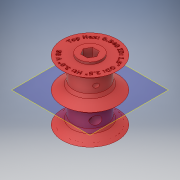
# Autodesk Inventor part: spoolV08
Saved by Autodesk Inventor 2019.4 (Build 234330000, 330)
## iProperties
Created: 2019-02-25
Part Number: spoolV08
Material: PC/ABS Plastic
Document SubType Name: Modeling
Designer: steele
Density: 0.357273 g/cm^3
Appearance: Smooth - Red
holeForString: 0.200 in
stringDiameter: 0.120 in
clearanceForString: 0.080 in
clearanceForHexShaft: 0.040 in
spoolInteriorDiameter: 1.500 in
spoolInteriroRadius: 0.750 in
spoolExteriorDiameter: 2.500 in
spoolExteriorRadius: 1.250 in
hexHoleChamfer: 0.063 in
stringHoleCenterFromHexShaft: 0.370 in
textCircleDiameter: 1.875 in
textHeight: 0.180 in
textDepth: 0.050 in
Author: steele
Autodesk Inventor part; units mm, degrees
(part 1 of 2)
ref_plane "XZ Plane" through (0, 0, 0) normal (0, 1, 0) x (-1, 0, 0)
sketch "Sketch15" plane through (0, 0, 0) normal (0, 0, 1) x (1, 0, 0)
  line L0 (31.75, 0) -> (31.75, 69.85) construction
  line L1 (12.065, 0) -> (31.75, 0)
  line L2 (13.335, 69.85) -> (31.75, 69.85)
  line L3 (19.05, 0) -> (19.05, 69.85) construction
  line L4 (0, 69.85) -> (0, 0)
  line L5 (19.05, 17.4625) -> (31.75, 17.4625) construction
  line L6 (31.75, 0) -> (19.05, 7.3323)
  line L7 (31.75, 34.925) -> (19.05, 27.5927)
  line L8 (19.05, 27.5927) -> (31.75, 27.5927) construction
  line L9 (19.05, 27.5927) -> (19.05, 7.3323)
  line L10 (31.75, 34.925) -> (19.05, 42.2573)
  line L11 (19.05, 42.2573) -> (19.05, 62.5177)
  line L12 (19.05, 62.5177) -> (31.75, 69.85)
  line L13 (31.75, 34.925) -> (19.05, 34.925) construction
  line L14 (19.05, 62.5177) -> (31.75, 62.5177) construction
  line L15 (0, 69.85) -> (0, 72.39)
  line L16 (0, 72.39) -> (13.335, 72.39)
  line L17 (13.335, 72.39) -> (13.335, 69.85)
  line L18 (0, 0) -> (0, -2.54)
  line L19 (0, -2.54) -> (12.065, -2.54)
  line L20 (12.065, -2.54) -> (12.065, 0)
  dimension "d85" = 31.75
  dimension "d86" = 69.85
  dimension "d87" = 19.05
  dimension "d88" = 31.75
  dimension "d89" = 34.925
  dimension "centerLineForSpool" = 17.4625
  dimension "d93" = 30
  dimension "d94" = 30
  dimension "d95" = 30
  dimension "d96" = 30
  dimension "d149" = 2.54
  dimension "d150" = 13.335
  dimension "d151" = 2.54
  dimension "d152" = 12.065
  constraints: 42 end point, 10 point on line, 5 perpendicular, 3 horizontal, 3 vertical, 2 midpoint, 1 collinear, 1 parallel
  measures "d85" distance from line of L4.end L0
  measures "d86" distance of L0.start L0.end
  measures "d87" distance from line of L3 L4.end
  measures "d88" distance of L4.start L0.end
  measures "d89" distance from line of L7.start L1
  measures "centerLineForSpool" distance from line of L5.start L1
  measures "d93" angle of L6 L1
  measures "d94" angle of L7 L8
  measures "d95" angle of L10 L13
  measures "d96" angle of L12 L14
  measures "d149" distance between parallel lines of L16 L2
  measures "d150" distance between parallel lines of L17 L15
  measures "d151" distance from line of L4.end L19
  measures "d152" distance between parallel lines of L20 L18
revolve "Revolution2" add sketch "Sketch15" angle 360 about axis through (0, 69.85, 0) along (0, -1, 0)
sketch "Sketch16" plane through (0, 0, 0) normal (0, -1, 0) x (1, 0, 0)
  line L0 (-7.9189, 0) -> (-3.9595, 6.858)
  line L1 (-3.9595, 6.858) -> (3.9595, 6.858)
  line L2 (3.9595, 6.858) -> (7.9189, 0)
  line L3 (7.9189, 0) -> (3.9595, -6.858)
  line L4 (3.9595, -6.858) -> (-3.9595, -6.858)
  line L5 (-3.9595, -6.858) -> (-7.9189, 0)
  point P0 (0, 0)
  point P1 (0, 0)
  dimension "d103" = 13.716
  constraints: 12 end point, 1 coincident, 1 horizontal, 13 other
  measures "d103" distance between parallel lines of L1 L4
extrude "Extrusion11" cut sketch "Sketch16" against normal through all
sketch "Sketch17" plane through (0, 0, 0) normal (1, 0, 0) x (0, 1, 0)
  circle A0 centre (52.3875, 9.398) radius 2.54
  circle A1 centre (17.4625, 9.398) radius 2.54
  line L0 (0, 31.75) -> (0, -31.75) projected
  line L1 (69.85, 31.75) -> (69.85, -31.75) projected
  line L2 (0, 6.858) -> (72.39, 6.858) projected
  point P0 (0, 0)
  point P1 (69.85, 6.858)
  dimension "d110" = 17.4625
  dimension "d111" = 17.4625
  dimension "d112" = 5.08
  constraints: 2 centre point, 2 tangent, 1 equal radius
  measures "d110" distance from line of A1.centre L0
  measures "d111" distance from line of A0.centre L1
  measures "d112" diameter of A0
extrude "Extrusion13" cut sketch "Sketch17" along normal through all both and the other way through all
ref_plane "Work Plane4" through (-19.05, 0, 0) normal (1, 0, 0) x (0, 1, 0)
sketch "Sketch22" plane through (-19.05, 0, 0) normal (1, 0, 0) x (0, 1, 0)
  spline S0 degree 7 poles (54.9275, 9.398) (54.9275, 9.7003) (54.8855, 9.9947) (54.8055, 10.2759) (54.6914, 10.5396) (54.547, 10.7823) (54.3764, 11.0012) (53.983, 11.3946) (53.7559, 11.5694) (53.5066, 11.7139) (53.24, 11.8248) (52.9612, 11.9) (52.6753, 11.938) (52.1137, 11.938) (51.8403, 11.9036) (51.5721, 11.8349) (51.3141, 11.7328) (51.0711, 11.5991) (50.848, 11.4367) (50.4419, 11.0554) (50.2585, 10.8324) (50.103, 10.5833) (49.9797, 10.311) (49.8931, 10.0193) (49.8475, 9.713) (49.8475, 9.1243) (49.8819, 8.8508) (49.9506, 8.5825) (50.0528, 8.3245) (50.1864, 8.0817) (50.3487, 7.8586) (50.7502, 7.431) (50.9916, 7.2397) (51.2531, 7.0865) (51.5286, 6.9719) (51.8128, 6.8958) (52.1007, 6.858) (52.7051, 6.858) (53.0247, 6.9043) (53.3394, 6.998) (53.642, 7.1395) (53.9245, 7.3282) (54.1787, 7.563) (54.5393, 8.0279) (54.6661, 8.2331) (54.7705, 8.4538) (54.8497, 8.6855) (54.9021, 8.9235) (54.9275, 9.1626) (54.9275, 9.398) knots 0 0 0 0 0 0 0 0 0.127217 0.127217 0.127217 0.127217 0.127217 0.127217 0.25952 0.25952 0.25952 0.25952 0.25952 0.25952 0.385403 0.385403 0.385403 0.385403 0.385403 0.385403 0.516079 0.516079 0.516079 0.516079 0.516079 0.516079 0.629606 0.629606 0.629606 0.629606 0.629606 0.629606 0.75956 0.75956 0.75956 0.75956 0.75956 0.75956 0.903464 0.903464 0.903464 0.903464 0.903464 0.903464 1 1 1 1 1 1 1 1 projected
  circle A0 centre (52.3875, 9.398) radius 4.7625
  circle A1 centre (52.3875, 9.398) radius 2.54 construction
  line L0 (52.3875, 6.858) -> (72.39, 6.858) construction
  line L1 (69.85, 31.75) -> (69.85, -31.75) construction
  point P0 (0, 0)
  point P1 (69.85, 6.858)
  dimension "d121" = 17.4625
  dimension "d122" = 5.08
  dimension "d125" = 9.525
  constraints: 2 centre point, 1 concentric, 1 tangent, 1 vertical alignment
  measures "d121" distance from line of A1.centre L1
  measures "d122" diameter of A1
  measures "d125" diameter of A0
extrude "Extrusion16" cut sketch "Sketch22" along normal blind 11.1125
ref_plane "Work Plane5" through (19.05, 0, 0) normal (1, 0, 0) x (0, 1, 0)
sketch "Sketch23" plane through (19.05, 0, 0) normal (1, 0, 0) x (0, 1, 0)
  line L0 (17.4625, 6.858) -> (52.3875, 6.858) projected
  circle A0 centre (17.4625, 9.398) radius 2.54 construction
  line L1 (0, 31.75) -> (0, -31.75) projected
  circle A1 centre (17.4625, 9.398) radius 4.7625
  point P0 (0, 0)
  dimension "d127" = 5.08
  dimension "d128" = 17.4625
  dimension "d129" = 9.525
  constraints: 2 centre point, 1 coincident, 1 tangent
  measures "d127" diameter of A0
  measures "d128" distance from line of A0.centre L1
  measures "d129" diameter of A1
extrude "Extrusion17" cut sketch "Sketch23" against normal blind 11.1125
chamfer "Chamfer12" distance 2.3813 angle 45 4 edges at (-19.05, 62.5177, 0) (-19.05, 42.2573, 0) (-19.05, 27.5927, 0) (-19.05, 7.3323, 0)
ref_plane "Work Plane6" through (0, 34.925, 0) normal (0, -1, 0) x (1, 0, 0)
sketch "Sketch24" plane through (0, 69.85, 0) normal (0, 1, 0) x (1, 0, 0)
  circle A0 centre (0, 0) radius 23.8125 construction
  line L0 (-23.7846, 1.2735) -> (-27.2701, 1.5398)
  line L1 (-27.2701, 1.5398) -> (-27.3674, 0.2663)
  line L2 (-27.3674, 0.2663) -> (-28.1874, 0.329)
  line L3 (-28.1874, 0.329) -> (-27.9101, 3.9576)
  line L4 (-27.9101, 3.9576) -> (-27.0902, 3.8949)
  line L5 (-27.0902, 3.8949) -> (-27.1875, 2.6214)
  line L6 (-27.1875, 2.6214) -> (-23.702, 2.3551)
  line L7 (-23.702, 2.3551) -> (-23.7846, 1.2735)
  spline S0 degree 2 poles (-24.3916, 7.4198) (-23.6078, 7.2369) (-22.9078, 6.1716) (-23.09, 5.3912) knots 0 0 0 1 2 2 2
  spline S1 degree 2 poles (-23.09, 5.3912) (-23.2713, 4.6143) (-24.3722, 3.9622) (-25.1559, 4.1451) knots 0 0 0 1 2 2 2
  spline S2 degree 2 poles (-25.1559, 4.1451) (-25.9465, 4.3296) (-26.6414, 5.4009) (-26.4601, 6.1779) knots 0 0 0 1 2 2 2
  spline S3 degree 2 poles (-26.4601, 6.1779) (-26.2788, 6.9548) (-25.1787, 7.6035) (-24.3916, 7.4198) knots 0 0 0 1 2 2 2
  spline S4 degree 2 poles (-24.621, 6.4061) (-24.9038, 6.4722) (-25.3035, 6.4684) (-25.4351, 6.4129) knots 0 0 0 1 2 2 2
  spline S5 degree 2 poles (-25.4351, 6.4129) (-25.575, 6.3521) (-25.7187, 6.1521) (-25.7513, 6.0124) knots 0 0 0 1 2 2 2
  spline S6 degree 2 poles (-25.7513, 6.0124) (-25.7831, 5.8761) (-25.7515, 5.6423) (-25.6563, 5.5267) knots 0 0 0 1 2 2 2
  spline S7 degree 2 poles (-25.6563, 5.5267) (-25.5671, 5.4161) (-25.2059, 5.224) (-24.9129, 5.1556) knots 0 0 0 1 2 2 2
  spline S8 degree 2 poles (-24.9129, 5.1556) (-24.6232, 5.088) (-24.2432, 5.0999) (-24.1158, 5.1528) knots 0 0 0 1 2 2 2
  spline S9 degree 2 poles (-24.1158, 5.1528) (-23.9885, 5.2057) (-23.8306, 5.4204) (-23.7972, 5.5635) knots 0 0 0 1 2 2 2
  spline S10 degree 2 poles (-23.7972, 5.5635) (-23.7693, 5.6828) (-23.8143, 5.952) (-23.899, 6.0508) knots 0 0 0 1 2 2 2
  spline S11 degree 2 poles (-23.899, 6.0508) (-23.9984, 6.1638) (-24.3211, 6.3362) (-24.621, 6.4061) knots 0 0 0 1 2 2 2
  spline S12 degree 2 poles (-22.9837, 11.143) (-22.2604, 10.8504) (-21.6713, 9.7591) (-21.8892, 9.2206) knots 0 0 0 1 2 2 2
  spline S13 degree 2 poles (-21.8892, 9.2206) (-21.9797, 8.9968) (-22.2154, 8.7033) (-22.4018, 8.5598) knots 0 0 0 1 2 2 2
  line L8 (-22.4018, 8.5598) -> (-21.1432, 8.0507)
  line L9 (-21.1432, 8.0507) -> (-21.5237, 7.1099)
  line L10 (-21.5237, 7.1099) -> (-25.6499, 8.779)
  line L11 (-25.6499, 8.779) -> (-25.2694, 9.7197)
  line L12 (-25.2694, 9.7197) -> (-24.9515, 9.5912)
  spline S14 degree 2 poles (-24.9515, 9.5912) (-25.0459, 9.8709) (-25.0933, 10.3883) (-24.9791, 10.6706) knots 0 0 0 1 2 2 2
  spline S15 degree 2 poles (-24.9791, 10.6706) (-24.7666, 11.1961) (-23.7006, 11.433) (-22.9837, 11.143) knots 0 0 0 1 2 2 2
  spline S16 degree 2 poles (-23.354, 10.1717) (-23.7952, 10.3502) (-24.3011, 10.2378) (-24.4166, 9.9523) knots 0 0 0 1 2 2 2
  spline S17 degree 2 poles (-24.4166, 9.9523) (-24.4678, 9.8258) (-24.4877, 9.5432) (-24.4552, 9.3904) knots 0 0 0 1 2 2 2
  line L13 (-24.4552, 9.3904) -> (-22.9403, 8.7776)
  spline S18 degree 2 poles (-22.9403, 8.7776) (-22.8777, 8.8391) (-22.7782, 9.0103) (-22.7284, 9.1335) knots 0 0 0 1 2 2 2
  spline S19 degree 2 poles (-22.7284, 9.1335) (-22.5906, 9.4741) (-22.9031, 9.9893) (-23.354, 10.1717) knots 0 0 0 1 2 2 2
  line L14 (-18.1571, 15.5136) -> (-18.7968, 14.6375)
  line L15 (-18.7968, 14.6375) -> (-20.3426, 15.7663)
  line L16 (-20.3426, 15.7663) -> (-21.2114, 14.5765)
  line L17 (-21.2114, 14.5765) -> (-19.6656, 13.4478)
  line L18 (-19.6656, 13.4478) -> (-20.3053, 12.5717)
  line L19 (-20.3053, 12.5717) -> (-23.7925, 15.1181)
  line L20 (-23.7925, 15.1181) -> (-23.1528, 15.9942)
  line L21 (-23.1528, 15.9942) -> (-21.8755, 15.0615)
  line L22 (-21.8755, 15.0615) -> (-21.0067, 16.2512)
  line L23 (-21.0067, 16.2512) -> (-22.2841, 17.1839)
  line L24 (-22.2841, 17.1839) -> (-21.6444, 18.06)
  line L25 (-21.6444, 18.06) -> (-18.1571, 15.5136)
  spline S20 degree 2 poles (-16.3247, 17.2183) (-16.9871, 16.5744) (-18.3068, 16.5215) (-18.875, 17.1061) knots 0 0 0 1 2 2 2
  spline S21 degree 2 poles (-18.875, 17.1061) (-19.4311, 17.6782) (-19.437, 18.9997) (-18.8448, 19.5753) knots 0 0 0 1 2 2 2
  spline S22 degree 2 poles (-18.8448, 19.5753) (-18.3103, 20.0948) (-17.205, 20.0419) (-16.6831, 19.5049) knots 0 0 0 1 2 2 2
  line L26 (-16.6831, 19.5049) -> (-16.427, 19.2414)
  line L27 (-16.427, 19.2414) -> (-18.0254, 17.6879)
  spline S23 degree 2 poles (-18.0254, 17.6879) (-17.8568, 17.5346) (-17.5292, 17.4334) (-17.3704, 17.4608) knots 0 0 0 1 2 2 2
  spline S24 degree 2 poles (-17.3704, 17.4608) (-17.2142, 17.4858) (-16.9096, 17.6745) (-16.7615, 17.8184) knots 0 0 0 1 2 2 2
  spline S25 degree 2 poles (-16.7615, 17.8184) (-16.6361, 17.9403) (-16.4438, 18.2345) (-16.3873, 18.3822) knots 0 0 0 1 2 2 2
  spline S26 degree 2 poles (-16.3873, 18.3822) (-16.3335, 18.5076) (-16.2732, 18.7468) (-16.2596, 18.8283) knots 0 0 0 1 2 2 2
  line L28 (-16.2596, 18.8283) -> (-16.1819, 18.9039)
  line L29 (-16.1819, 18.9039) -> (-15.5965, 18.3016)
  spline S27 degree 2 poles (-15.5965, 18.3016) (-15.6527, 18.1787) (-15.7397, 17.977) (-15.841, 17.8201) knots 0 0 0 1 2 2 2
  spline S28 degree 2 poles (-15.841, 17.8201) (-15.9272, 17.6729) (-16.144, 17.3939) (-16.3247, 17.2183) knots 0 0 0 1 2 2 2
  spline S29 degree 2 poles (-17.5714, 18.9831) (-17.8008, 19.209) (-18.2406, 19.2549) (-18.4489, 19.0525) knots 0 0 0 1 2 2 2
  spline S30 degree 2 poles (-18.4489, 19.0525) (-18.6622, 18.8452) (-18.6543, 18.3551) (-18.4547, 18.1246) knots 0 0 0 1 2 2 2
  line L30 (-18.4547, 18.1246) -> (-17.5714, 18.9831)
  line L31 (-12.4065, 20.4043) -> (-13.3737, 19.7116)
  line L32 (-13.3737, 19.7116) -> (-14.4212, 20.1105)
  line L33 (-14.4212, 20.1105) -> (-14.395, 18.9801)
  line L34 (-14.395, 18.9801) -> (-15.3423, 18.3016)
  line L35 (-15.3423, 18.3016) -> (-15.316, 20.3261)
  line L36 (-15.316, 20.3261) -> (-17.2222, 20.9623)
  line L37 (-17.2222, 20.9623) -> (-16.2549, 21.6551)
  line L38 (-16.2549, 21.6551) -> (-15.2261, 21.2643)
  line L39 (-15.2261, 21.2643) -> (-15.2621, 22.3662)
  line L40 (-15.2621, 22.3662) -> (-14.3148, 23.0447)
  line L41 (-14.3148, 23.0447) -> (-14.3403, 21.0551)
  line L42 (-14.3403, 21.0551) -> (-12.4065, 20.4043)
  line L43 (-11.9945, 22.9943) -> (-12.8939, 22.5022)
  line L44 (-12.8939, 22.5022) -> (-13.4415, 23.5029)
  line L45 (-13.4415, 23.5029) -> (-12.542, 23.995)
  line L46 (-12.542, 23.995) -> (-11.9945, 22.9943)
  line L47 (-10.9784, 21.1371) -> (-11.8778, 20.645)
  line L48 (-11.8778, 20.645) -> (-12.4253, 21.6457)
  line L49 (-12.4253, 21.6457) -> (-11.5259, 22.1378)
  line L50 (-11.5259, 22.1378) -> (-10.9784, 21.1371)
  spline S31 degree 2 poles (-6.1652, 25.2839) (-5.998, 24.7496) (-5.9177, 23.8948) (-6.0234, 23.5648) knots 0 0 0 1 2 2 2
  spline S32 degree 2 poles (-6.0234, 23.5648) (-6.1269, 23.2391) (-6.6457, 22.7762) (-7.0798, 22.6404) knots 0 0 0 1 2 2 2
  spline S33 degree 2 poles (-7.0798, 22.6404) (-7.5173, 22.5035) (-8.2041, 22.5894) (-8.4801, 22.8037) knots 0 0 0 1 2 2 2
  spline S34 degree 2 poles (-8.4801, 22.8037) (-8.7551, 23.0146) (-9.174, 23.7562) (-9.3412, 24.2905) knots 0 0 0 1 2 2 2
  spline S35 degree 2 poles (-9.3412, 24.2905) (-9.5125, 24.8382) (-9.5845, 25.6663) (-9.4786, 26.0074) knots 0 0 0 1 2 2 2
  spline S36 degree 2 poles (-9.4786, 26.0074) (-9.3705, 26.3419) (-8.8429, 26.8002) (-8.4221, 26.9318) knots 0 0 0 1 2 2 2
  spline S37 degree 2 poles (-8.4221, 26.9318) (-7.978, 27.0707) (-7.2958, 26.9761) (-7.0187, 26.7585) knots 0 0 0 1 2 2 2
  spline S38 degree 2 poles (-7.0187, 26.7585) (-6.7471, 26.5465) (-6.3271, 25.8016) (-6.1652, 25.2839) knots 0 0 0 1 2 2 2
  spline S39 degree 2 poles (-7.2038, 24.9591) (-7.443, 25.7239) (-7.8867, 26.2633) (-8.184, 26.1704) knots 0 0 0 1 2 2 2
  spline S40 degree 2 poles (-8.184, 26.1704) (-8.4812, 26.0774) (-8.5418, 25.3802) (-8.3015, 24.6121) knots 0 0 0 1 2 2 2
  spline S41 degree 2 poles (-8.3015, 24.6121) (-8.0654, 23.8573) (-7.6152, 23.3088) (-7.318, 23.4018) knots 0 0 0 1 2 2 2
  spline S42 degree 2 poles (-7.318, 23.4018) (-7.0241, 23.4937) (-6.9667, 24.201) (-7.2038, 24.9591) knots 0 0 0 1 2 2 2
  line L51 (-3.8773, 23.5003) -> (-4.8851, 23.3117)
  line L52 (-4.8851, 23.3117) -> (-5.0949, 24.433)
  line L53 (-5.0949, 24.433) -> (-4.0871, 24.6215)
  line L54 (-4.0871, 24.6215) -> (-3.8773, 23.5003)
  spline S43 degree 2 poles (-0.0685, 25.3271) (-0.0459, 24.9884) (-0.238, 24.4004) (-0.4512, 24.1792) knots 0 0 0 1 2 2 2
  spline S44 degree 2 poles (-0.4512, 24.1792) (-0.6644, 23.958) (-1.2706, 23.6895) (-1.7245, 23.6592) knots 0 0 0 1 2 2 2
  spline S45 degree 2 poles (-1.7245, 23.6592) (-2.2066, 23.6304) (-2.9084, 23.7413) (-3.1421, 23.8274) knots 0 0 0 1 2 2 2
  line L55 (-3.1421, 23.8274) -> (-3.2049, 24.7666)
  line L56 (-3.2049, 24.7666) -> (-3.1071, 24.7731)
  spline S46 degree 2 poles (-3.1071, 24.7731) (-3.0203, 24.7333) (-2.8099, 24.6282) (-2.6416, 24.5763) knots 0 0 0 1 2 2 2
  spline S47 degree 2 poles (-2.6416, 24.5763) (-2.484, 24.5272) (-2.1609, 24.4682) (-1.9689, 24.481) knots 0 0 0 1 2 2 2
  spline S48 degree 2 poles (-1.9689, 24.481) (-1.8013, 24.4922) (-1.4159, 24.6022) (-1.3046, 24.7218) knots 0 0 0 1 2 2 2
  spline S49 degree 2 poles (-1.3046, 24.7218) (-1.2232, 24.815) (-1.1397, 25.0345) (-1.1516, 25.2125) knots 0 0 0 1 2 2 2
  spline S50 degree 2 poles (-1.1516, 25.2125) (-1.1618, 25.3661) (-1.302, 25.5742) (-1.4077, 25.6338) knots 0 0 0 1 2 2 2
  spline S51 degree 2 poles (-1.4077, 25.6338) (-1.5609, 25.7217) (-1.9836, 25.7496) (-2.1337, 25.7395) knots 0 0 0 1 2 2 2
  spline S52 degree 2 poles (-2.1337, 25.7395) (-2.3711, 25.7236) (-2.8164, 25.6167) (-2.9777, 25.5638) knots 0 0 0 1 2 2 2
  line L57 (-2.9777, 25.5638) -> (-3.0719, 25.5575)
  line L58 (-3.0719, 25.5575) -> (-3.2338, 27.9771)
  line L59 (-3.2338, 27.9771) -> (-0.3778, 28.1681)
  line L60 (-0.3778, 28.1681) -> (-0.3234, 27.3546)
  line L61 (-0.3234, 27.3546) -> (-2.1564, 27.232)
  line L62 (-2.1564, 27.232) -> (-2.1085, 26.5163)
  spline S53 degree 2 poles (-2.1085, 26.5163) (-2.0217, 26.5291) (-1.7813, 26.5522) (-1.7149, 26.5566) knots 0 0 0 1 2 2 2
  spline S54 degree 2 poles (-1.7149, 26.5566) (-1.4042, 26.5774) (-0.8721, 26.4867) (-0.6574, 26.3713) knots 0 0 0 1 2 2 2
  spline S55 degree 2 poles (-0.6574, 26.3713) (-0.4023, 26.2271) (-0.0942, 25.7111) (-0.0685, 25.3271) knots 0 0 0 1 2 2 2
  line L63 (4.0385, 24.5536) -> (3.4566, 24.6071)
  line L64 (3.4566, 24.6071) -> (3.3633, 23.5931)
  line L65 (3.3633, 23.5931) -> (2.3214, 23.689)
  line L66 (2.3214, 23.689) -> (2.4147, 24.7029)
  line L67 (2.4147, 24.7029) -> (0.5191, 24.8773)
  line L68 (0.5191, 24.8773) -> (0.5929, 25.6787)
  line L69 (0.5929, 25.6787) -> (2.6831, 28.0025)
  line L70 (2.6831, 28.0025) -> (3.7598, 27.9034)
  line L71 (3.7598, 27.9034) -> (3.5277, 25.3806)
  line L72 (3.5277, 25.3806) -> (4.1096, 25.3271)
  line L73 (4.1096, 25.3271) -> (4.0385, 24.5536)
  line L74 (2.4859, 25.4765) -> (2.6205, 26.94)
  line L75 (2.6205, 26.94) -> (1.3952, 25.5768)
  line L76 (1.3952, 25.5768) -> (2.4859, 25.4765)
  spline S56 degree 2 poles (8.0437, 24.7505) (7.9051, 24.208) (7.5242, 23.4386) (7.2608, 23.2134) knots 0 0 0 1 2 2 2
  spline S57 degree 2 poles (7.2608, 23.2134) (7.0016, 22.9907) (6.3169, 22.8695) (5.8762, 22.9822) knots 0 0 0 1 2 2 2
  spline S58 degree 2 poles (5.8762, 22.9822) (5.4321, 23.0957) (4.8929, 23.5297) (4.7707, 23.8571) knots 0 0 0 1 2 2 2
  spline S59 degree 2 poles (4.7707, 23.8571) (4.6477, 24.1811) (4.681, 25.0321) (4.8197, 25.5746) knots 0 0 0 1 2 2 2
  spline S60 degree 2 poles (4.8197, 25.5746) (4.9618, 26.1306) (5.3357, 26.8729) (5.6051, 27.1074) knots 0 0 0 1 2 2 2
  spline S61 degree 2 poles (5.6051, 27.1074) (5.8728, 27.3351) (6.5625, 27.4478) (6.9897, 27.3386) knots 0 0 0 1 2 2 2
  spline S62 degree 2 poles (6.9897, 27.3386) (7.4406, 27.2233) (7.9713, 26.7843) (8.0926, 26.4535) knots 0 0 0 1 2 2 2
  spline S63 degree 2 poles (8.0926, 26.4535) (8.2122, 26.1304) (8.178, 25.2759) (8.0437, 24.7505) knots 0 0 0 1 2 2 2
  spline S64 degree 2 poles (6.9894, 25.02) (7.1878, 25.7963) (7.0939, 26.4885) (6.7921, 26.5656) knots 0 0 0 1 2 2 2
  spline S65 degree 2 poles (6.7921, 26.5656) (6.4904, 26.6427) (6.0724, 26.0814) (5.8731, 25.3017) knots 0 0 0 1 2 2 2
  spline S66 degree 2 poles (5.8731, 25.3017) (5.6773, 24.5355) (5.772, 23.8323) (6.0738, 23.7552) knots 0 0 0 1 2 2 2
  spline S67 degree 2 poles (6.0738, 23.7552) (6.3721, 23.6789) (6.7927, 24.2504) (6.9894, 25.02) knots 0 0 0 1 2 2 2
  line L77 (11.6683, 20.7903) -> (9.5891, 21.8274)
  line L78 (9.5891, 21.8274) -> (9.9249, 22.5006)
  line L79 (9.9249, 22.5006) -> (10.4792, 22.2241)
  line L80 (10.4792, 22.2241) -> (11.7349, 24.7417)
  line L81 (11.7349, 24.7417) -> (11.1807, 25.0181)
  line L82 (11.1807, 25.0181) -> (11.5165, 25.6913)
  line L83 (11.5165, 25.6913) -> (13.5956, 24.6543)
  line L84 (13.5956, 24.6543) -> (13.2598, 23.981)
  line L85 (13.2598, 23.981) -> (12.7056, 24.2575)
  line L86 (12.7056, 24.2575) -> (11.4499, 21.7399)
  line L87 (11.4499, 21.7399) -> (12.0041, 21.4635)
  line L88 (12.0041, 21.4635) -> (11.6683, 20.7903)
  spline S68 degree 2 poles (16.6986, 19.9926) (16.3483, 19.4989) (15.3667, 19.0283) (14.8907, 19.0528) knots 0 0 0 1 2 2 2
  spline S69 degree 2 poles (14.8907, 19.0528) (14.4912, 19.0702) (13.7733, 19.425) (13.4108, 19.6822) knots 0 0 0 1 2 2 2
  line L89 (13.4108, 19.6822) -> (12.3092, 20.4636)
  line L90 (12.3092, 20.4636) -> (14.8075, 23.9855)
  line L91 (14.8075, 23.9855) -> (15.8977, 23.2121)
  spline S70 degree 2 poles (15.8977, 23.2121) (16.2688, 22.9489) (16.8498, 22.3951) (17.0056, 22.01) knots 0 0 0 1 2 2 2
  spline S71 degree 2 poles (17.0056, 22.01) (17.1931, 21.5424) (17.061, 20.5035) (16.6986, 19.9926) knots 0 0 0 1 2 2 2
  spline S72 degree 2 poles (15.7951, 20.6422) (16.0421, 20.9904) (16.1546, 21.657) (16.0084, 21.971) knots 0 0 0 1 2 2 2
  spline S73 degree 2 poles (16.0084, 21.971) (15.8974, 22.1956) (15.5177, 22.4949) (15.2437, 22.6893) knots 0 0 0 1 2 2 2
  line L92 (15.2437, 22.6893) -> (15.2266, 22.7014)
  line L93 (15.2266, 22.7014) -> (13.6616, 20.4953)
  line L94 (13.6616, 20.4953) -> (13.6787, 20.4831)
  spline S74 degree 2 poles (13.6787, 20.4831) (13.9755, 20.2726) (14.3978, 20.0031) (14.6664, 19.9885) knots 0 0 0 1 2 2 2
  spline S75 degree 2 poles (14.6664, 19.9885) (14.9804, 19.9716) (15.5481, 20.294) (15.7951, 20.6422) knots 0 0 0 1 2 2 2
  line L95 (18.1689, 18.5066) -> (17.4232, 19.2102)
  line L96 (17.4232, 19.2102) -> (18.2061, 20.0399)
  line L97 (18.2061, 20.0399) -> (18.9518, 19.3363)
  line L98 (18.9518, 19.3363) -> (18.1689, 18.5066)
  line L99 (16.7161, 16.9668) -> (15.9704, 17.6704)
  line L100 (15.9704, 17.6704) -> (16.7532, 18.5001)
  line L101 (16.7532, 18.5001) -> (17.4989, 17.7965)
  line L102 (17.4989, 17.7965) -> (16.7161, 16.9668)
  line L103 (20.3063, 12.5309) -> (18.6563, 14.857)
  line L104 (18.6563, 14.857) -> (19.27, 15.2923)
  line L105 (19.27, 15.2923) -> (19.7963, 14.5502)
  line L106 (19.7963, 14.5502) -> (21.66, 15.8722)
  line L107 (21.66, 15.8722) -> (21.1337, 16.6142)
  line L108 (21.1337, 16.6142) -> (21.7074, 17.0212)
  spline S76 degree 2 poles (21.7074, 17.0212) (21.8227, 16.8585) (22.0943, 16.5663) (22.2088, 16.5017) knots 0 0 0 1 2 2 2
  spline S77 degree 2 poles (22.2088, 16.5017) (22.3449, 16.4309) (22.6252, 16.4409) (22.776, 16.5307) knots 0 0 0 1 2 2 2
  line L109 (22.776, 16.5307) -> (23.3226, 15.7601)
  line L110 (23.3226, 15.7601) -> (20.4057, 13.6911)
  line L111 (20.4057, 13.6911) -> (20.9199, 12.9662)
  line L112 (20.9199, 12.9662) -> (20.3063, 12.5309)
  line L113 (21.1558, 10.942) -> (20.6654, 11.8423)
  line L114 (20.6654, 11.8423) -> (21.6672, 12.388)
  line L115 (21.6672, 12.388) -> (22.1576, 11.4876)
  line L116 (22.1576, 11.4876) -> (21.1558, 10.942)
  spline S78 degree 2 poles (24.0691, 7.8831) (23.754, 7.757) (23.1354, 7.7583) (22.8592, 7.8928) knots 0 0 0 1 2 2 2
  spline S79 degree 2 poles (22.8592, 7.8928) (22.583, 8.0272) (22.1405, 8.521) (21.9715, 8.9434) knots 0 0 0 1 2 2 2
  spline S80 degree 2 poles (21.9715, 8.9434) (21.7954, 9.393) (21.6842, 10.0948) (21.6939, 10.3436) knots 0 0 0 1 2 2 2
  line L117 (21.6939, 10.3436) -> (22.5679, 10.6933)
  line L118 (22.5679, 10.6933) -> (22.6042, 10.6023)
  spline S81 degree 2 poles (22.6042, 10.6023) (22.5932, 10.5075) (22.5581, 10.2748) (22.5608, 10.0987) knots 0 0 0 1 2 2 2
  spline S82 degree 2 poles (22.5608, 10.0987) (22.5627, 9.9337) (22.6063, 9.6082) (22.6778, 9.4295) knots 0 0 0 1 2 2 2
  spline S83 degree 2 poles (22.6778, 9.4295) (22.7402, 9.2735) (22.9637, 8.9409) (23.1119, 8.872) knots 0 0 0 1 2 2 2
  spline S84 degree 2 poles (23.1119, 8.872) (23.2256, 8.8233) (23.4602, 8.8116) (23.6258, 8.8779) knots 0 0 0 1 2 2 2
  spline S85 degree 2 poles (23.6258, 8.8779) (23.7688, 8.9351) (23.9234, 9.1326) (23.9475, 9.2515) knots 0 0 0 1 2 2 2
  spline S86 degree 2 poles (23.9475, 9.2515) (23.9838, 9.4244) (23.8798, 9.835) (23.8239, 9.9747) knots 0 0 0 1 2 2 2
  spline S87 degree 2 poles (23.8239, 9.9747) (23.7356, 10.1957) (23.4964, 10.5862) (23.3963, 10.7233) knots 0 0 0 1 2 2 2
  line L119 (23.3963, 10.7233) -> (23.3612, 10.811)
  line L120 (23.3612, 10.811) -> (25.6126, 11.7118)
  line L121 (25.6126, 11.7118) -> (26.6759, 9.0542)
  line L122 (26.6759, 9.0542) -> (25.9189, 8.7514)
  line L123 (25.9189, 8.7514) -> (25.2365, 10.457)
  line L124 (25.2365, 10.457) -> (24.5705, 10.1905)
  spline S88 degree 2 poles (24.5705, 10.1905) (24.6095, 10.1119) (24.7057, 9.8903) (24.7304, 9.8286) knots 0 0 0 1 2 2 2
  spline S89 degree 2 poles (24.7304, 9.8286) (24.8461, 9.5395) (24.9241, 9.0054) (24.8806, 8.7656) knots 0 0 0 1 2 2 2
  spline S90 degree 2 poles (24.8806, 8.7656) (24.8221, 8.4784) (24.4265, 8.0261) (24.0691, 7.8831) knots 0 0 0 1 2 2 2
  line L125 (27.475, 6.88) -> (25.7748, 6.6434)
  line L126 (25.7748, 6.6434) -> (25.6332, 7.2211)
  line L127 (25.6332, 7.2211) -> (27.25, 7.7976)
  line L128 (27.25, 7.7976) -> (27.475, 6.88)
  line L129 (27.7658, 5.6939) -> (26.0656, 5.4573)
  line L130 (26.0656, 5.4573) -> (25.924, 6.035)
  line L131 (25.924, 6.035) -> (27.5408, 6.6116)
  line L132 (27.5408, 6.6116) -> (27.7658, 5.6939)
  spline S91 degree 2 poles (25.9925, -1.8107) (24.9428, -1.822) (23.7306, -0.7153) (23.7201, 0.2574) knots 0 0 0 1 2 2 2
  spline S92 degree 2 poles (23.7201, 0.2574) (23.7096, 1.2336) (24.9118, 2.3594) (25.9475, 2.3706) knots 0 0 0 1 2 2 2
  spline S93 degree 2 poles (25.9475, 2.3706) (26.9867, 2.3818) (28.2093, 1.2822) (28.2198, 0.3059) knots 0 0 0 1 2 2 2
  spline S94 degree 2 poles (28.2198, 0.3059) (28.2303, -0.6668) (27.0387, -1.7994) (25.9925, -1.8107) knots 0 0 0 1 2 2 2
  spline S95 degree 2 poles (25.9805, -0.691) (26.3688, -0.6868) (26.9095, -0.5235) (27.0795, -0.3852) knots 0 0 0 1 2 2 2
  spline S96 degree 2 poles (27.0795, -0.3852) (27.2564, -0.2469) (27.4066, 0.1047) (27.4046, 0.2936) knots 0 0 0 1 2 2 2
  spline S97 degree 2 poles (27.4046, 0.2936) (27.4024, 0.4931) (27.2555, 0.8169) (27.0719, 0.9654) knots 0 0 0 1 2 2 2
  spline S98 degree 2 poles (27.0719, 0.9654) (26.9025, 1.0966) (26.3444, 1.2551) (25.9595, 1.2509) knots 0 0 0 1 2 2 2
  spline S99 degree 2 poles (25.9595, 1.2509) (25.5606, 1.2466) (25.0375, 1.0835) (24.8605, 0.9451) knots 0 0 0 1 2 2 2
  spline S100 degree 2 poles (24.8605, 0.9451) (24.6835, 0.8067) (24.5334, 0.4517) (24.5354, 0.2627) knots 0 0 0 1 2 2 2
  spline S101 degree 2 poles (24.5354, 0.2627) (24.5375, 0.0703) (24.7058, -0.2848) (24.8821, -0.4124) knots 0 0 0 1 2 2 2
  spline S102 degree 2 poles (24.8821, -0.4124) (25.0726, -0.5503) (25.5746, -0.6954) (25.9805, -0.691) knots 0 0 0 1 2 2 2
  spline S103 degree 2 poles (25.1871, -6.6453) (24.5914, -6.5375) (23.749, -5.848) (23.5693, -5.4065) knots 0 0 0 1 2 2 2
  spline S104 degree 2 poles (23.5693, -5.4065) (23.4157, -5.0373) (23.4326, -4.2367) (23.5117, -3.7994) knots 0 0 0 1 2 2 2
  line L133 (23.5117, -3.7994) -> (23.7523, -2.4703)
  line L134 (23.7523, -2.4703) -> (28.0013, -3.2395)
  line L135 (28.0013, -3.2395) -> (27.7632, -4.5549)
  spline S105 degree 2 poles (27.7632, -4.5549) (27.6821, -5.0025) (27.427, -5.7635) (27.1443, -6.0679) knots 0 0 0 1 2 2 2
  spline S106 degree 2 poles (27.1443, -6.0679) (26.8003, -6.436) (25.8034, -6.7569) (25.1871, -6.6453) knots 0 0 0 1 2 2 2
  spline S107 degree 2 poles (25.3922, -5.5516) (25.8123, -5.6277) (26.4637, -5.4469) (26.6861, -5.1813) knots 0 0 0 1 2 2 2
  spline S108 degree 2 poles (26.6861, -5.1813) (26.8424, -4.9856) (26.9525, -4.5148) (27.0124, -4.1842) knots 0 0 0 1 2 2 2
  line L136 (27.0124, -4.1842) -> (27.0161, -4.1636)
  line L137 (27.0161, -4.1636) -> (24.3545, -3.6817)
  line L138 (24.3545, -3.6817) -> (24.3508, -3.7024)
  spline S109 degree 2 poles (24.3508, -3.7024) (24.2859, -4.0605) (24.2209, -4.5572) (24.3215, -4.8066) knots 0 0 0 1 2 2 2
  spline S110 degree 2 poles (24.3215, -4.8066) (24.4394, -5.0982) (24.9721, -5.4756) (25.3922, -5.5516) knots 0 0 0 1 2 2 2
  line L139 (24.4647, -8.6071) -> (24.7857, -7.6334)
  line L140 (24.7857, -7.6334) -> (25.8691, -7.9905)
  line L141 (25.8691, -7.9905) -> (25.5481, -8.9642)
  line L142 (25.5481, -8.9642) -> (24.4647, -8.6071)
  line L143 (22.4541, -7.9442) -> (22.7752, -6.9705)
  line L144 (22.7752, -6.9705) -> (23.8585, -7.3277)
  line L145 (23.8585, -7.3277) -> (23.5375, -8.3014)
  line L146 (23.5375, -8.3014) -> (22.4541, -7.9442)
  line L147 (19.8643, -13.244) -> (21.4301, -10.4834)
  line L148 (21.4301, -10.4834) -> (22.0418, -10.8304)
  spline S111 degree 2 poles (22.0418, -10.8304) (22.1233, -11.3393) (22.2988, -12.179) (22.4018, -12.515) knots 0 0 0 1 2 2 2
  spline S112 degree 2 poles (22.4018, -12.515) (22.5339, -12.956) (22.8354, -13.4528) (23.0667, -13.584) knots 0 0 0 1 2 2 2
  spline S113 degree 2 poles (23.0667, -13.584) (23.3285, -13.7325) (23.7863, -13.5778) (23.9451, -13.2978) knots 0 0 0 1 2 2 2
  spline S114 degree 2 poles (23.9451, -13.2978) (24.0263, -13.1548) (24.1013, -12.8594) (24.1207, -12.6974) knots 0 0 0 1 2 2 2
  spline S115 degree 2 poles (24.1207, -12.6974) (24.1354, -12.5368) (24.1172, -12.2851) (24.1127, -12.2222) knots 0 0 0 1 2 2 2
  line L149 (24.1127, -12.2222) -> (24.1541, -12.1492)
  line L150 (24.1541, -12.1492) -> (24.9729, -12.6135)
  spline S116 degree 2 poles (24.9729, -12.6135) (24.9592, -12.815) (24.7342, -13.5804) (24.5564, -13.8939) knots 0 0 0 1 2 2 2
  spline S117 degree 2 poles (24.5564, -13.8939) (24.1766, -14.5636) (23.1899, -14.9131) (22.6511, -14.6075) knots 0 0 0 1 2 2 2
  spline S118 degree 2 poles (22.6511, -14.6075) (22.3194, -14.4193) (21.858, -13.7433) (21.6982, -13.1739) knots 0 0 0 1 2 2 2
  spline S119 degree 2 poles (21.6982, -13.1739) (21.6025, -12.8179) (21.4958, -12.1902) (21.4763, -12.0544) knots 0 0 0 1 2 2 2
  line L151 (21.4763, -12.0544) -> (20.5734, -13.6463)
  line L152 (20.5734, -13.6463) -> (19.8643, -13.244)
  line L153 (18.8804, -14.5198) -> (19.4879, -13.6939)
  line L154 (19.4879, -13.6939) -> (20.4068, -14.3697)
  line L155 (20.4068, -14.3697) -> (19.7994, -15.1957)
  line L156 (19.7994, -15.1957) -> (18.8804, -14.5198)
  spline S120 degree 2 poles (17.3455, -18.4553) (17.0977, -18.2233) (16.8365, -17.6626) (16.8412, -17.3554) knots 0 0 0 1 2 2 2
  spline S121 degree 2 poles (16.8412, -17.3554) (16.8459, -17.0483) (17.1054, -16.4381) (17.4163, -16.106) knots 0 0 0 1 2 2 2
  spline S122 degree 2 poles (17.4163, -16.106) (17.7488, -15.7558) (18.3372, -15.3576) (18.5667, -15.2609) knots 0 0 0 1 2 2 2
  line L157 (18.5667, -15.2609) -> (19.254, -15.9041)
  line L158 (19.254, -15.9041) -> (19.187, -15.9756)
  spline S123 degree 2 poles (19.187, -15.9756) (19.0964, -16.0058) (18.8709, -16.0727) (18.7125, -16.1497) knots 0 0 0 1 2 2 2
  spline S124 degree 2 poles (18.7125, -16.1497) (18.5639, -16.2215) (18.2875, -16.399) (18.156, -16.5395) knots 0 0 0 1 2 2 2
  spline S125 degree 2 poles (18.156, -16.5395) (18.0412, -16.6621) (17.8348, -17.0057) (17.8352, -17.1691) knots 0 0 0 1 2 2 2
  spline S126 degree 2 poles (17.8352, -17.1691) (17.8393, -17.2927) (17.9282, -17.5101) (18.0585, -17.632) knots 0 0 0 1 2 2 2
  spline S127 degree 2 poles (18.0585, -17.632) (18.1709, -17.7372) (18.4154, -17.7935) (18.5333, -17.7649) knots 0 0 0 1 2 2 2
  spline S128 degree 2 poles (18.5333, -17.7649) (18.7052, -17.7245) (19.033, -17.4562) (19.1358, -17.3463) knots 0 0 0 1 2 2 2
  spline S129 degree 2 poles (19.1358, -17.3463) (19.2984, -17.1726) (19.5507, -16.7904) (19.6324, -16.6417) knots 0 0 0 1 2 2 2
  line L159 (19.6324, -16.6417) -> (19.697, -16.5727)
  line L160 (19.697, -16.5727) -> (21.4674, -18.2297)
  line L161 (21.4674, -18.2297) -> (19.5115, -20.3195)
  line L162 (19.5115, -20.3195) -> (18.9163, -19.7624)
  line L163 (18.9163, -19.7624) -> (20.1716, -18.4211)
  line L164 (20.1716, -18.4211) -> (19.6479, -17.931)
  spline S130 degree 2 poles (19.6479, -17.931) (19.5932, -17.9996) (19.4333, -18.1807) (19.3879, -18.2292) knots 0 0 0 1 2 2 2
  spline S131 degree 2 poles (19.3879, -18.2292) (19.1751, -18.4566) (18.7244, -18.7537) (18.4888, -18.816) knots 0 0 0 1 2 2 2
  spline S132 degree 2 poles (18.4888, -18.816) (18.2039, -18.8849) (17.6266, -18.7183) (17.3455, -18.4553) knots 0 0 0 1 2 2 2
  line L165 (17.8813, -21.9651) -> (16.9461, -20.5258)
  line L166 (16.9461, -20.5258) -> (17.4092, -20.1525)
  line L167 (17.4092, -20.1525) -> (18.617, -21.3723)
  line L168 (18.617, -21.3723) -> (17.8813, -21.9651)
  line L169 (16.9305, -22.7314) -> (15.9952, -21.2921)
  line L170 (15.9952, -21.2921) -> (16.4584, -20.9188)
  line L171 (16.4584, -20.9188) -> (17.6661, -22.1386)
  line L172 (17.6661, -22.1386) -> (16.9305, -22.7314)
  line L173 (8.7044, -22.2393) -> (9.6815, -21.768)
  line L174 (9.6815, -21.768) -> (10.513, -23.492)
  line L175 (10.513, -23.492) -> (11.8399, -22.852)
  line L176 (11.8399, -22.852) -> (11.0083, -21.128)
  line L177 (11.0083, -21.128) -> (11.9854, -20.6568)
  line L178 (11.9854, -20.6568) -> (13.8613, -24.546)
  line L179 (13.8613, -24.546) -> (12.8842, -25.0173)
  line L180 (12.8842, -25.0173) -> (12.1971, -23.5927)
  line L181 (12.1971, -23.5927) -> (10.8702, -24.2327)
  line L182 (10.8702, -24.2327) -> (11.5573, -25.6573)
  line L183 (11.5573, -25.6573) -> (10.5803, -26.1285)
  line L184 (10.5803, -26.1285) -> (8.7044, -22.2393)
  spline S133 degree 2 poles (6.696, -22.7895) (7.2872, -22.6049) (7.9806, -22.9237) (8.1537, -23.4781) knots 0 0 0 1 2 2 2
  line L185 (8.1537, -23.4781) -> (8.6074, -24.9311)
  line L186 (8.6074, -24.9311) -> (8.9782, -24.8153)
  line L187 (8.9782, -24.8153) -> (9.1888, -25.49)
  line L188 (9.1888, -25.49) -> (8.8181, -25.6058)
  line L189 (8.8181, -25.6058) -> (9.0955, -26.4943)
  line L190 (9.0955, -26.4943) -> (8.1268, -26.7967)
  line L191 (8.1268, -26.7967) -> (7.8494, -25.9082)
  line L192 (7.8494, -25.9082) -> (6.9142, -26.2003)
  line L193 (6.9142, -26.2003) -> (6.7035, -25.5256)
  line L194 (6.7035, -25.5256) -> (7.6388, -25.2335)
  line L195 (7.6388, -25.2335) -> (7.2935, -24.1279)
  spline S134 degree 2 poles (7.2935, -24.1279) (7.2424, -23.9643) (7.1596, -23.7225) (7.0893, -23.6382) knots 0 0 0 1 2 2 2
  spline S135 degree 2 poles (7.0893, -23.6382) (7.019, -23.5538) (6.7864, -23.5018) (6.5994, -23.5602) knots 0 0 0 1 2 2 2
  spline S136 degree 2 poles (6.5994, -23.5602) (6.5192, -23.5852) (6.2896, -23.7303) (6.2478, -23.7726) knots 0 0 0 1 2 2 2
  line L196 (6.2478, -23.7726) -> (6.1643, -23.7987)
  line L197 (6.1643, -23.7987) -> (5.9516, -23.1173)
  spline S137 degree 2 poles (5.9516, -23.1173) (6.096, -23.0282) (6.4355, -22.8709) (6.696, -22.7895) knots 0 0 0 1 2 2 2
  line L198 (4.7917, -25.4881) -> (5.7954, -25.2787)
  line L199 (5.7954, -25.2787) -> (6.0283, -26.3954)
  line L200 (6.0283, -26.3954) -> (5.0247, -26.6048)
  line L201 (5.0247, -26.6048) -> (4.7917, -25.4881)
  line L202 (4.3594, -23.4157) -> (5.363, -23.2063)
  line L203 (5.363, -23.2063) -> (5.596, -24.323)
  line L204 (5.596, -24.323) -> (4.5923, -24.5324)
  line L205 (4.5923, -24.5324) -> (4.3594, -23.4157)
  spline S138 degree 2 poles (-1.4059, -25.1335) (-1.4085, -24.8151) (-1.1784, -24.2918) (-0.9524, -24.108) knots 0 0 0 1 2 2 2
  spline S139 degree 2 poles (-0.9524, -24.108) (-0.7265, -23.9242) (-0.1087, -23.7232) (0.3357, -23.7196) knots 0 0 0 1 2 2 2
  spline S140 degree 2 poles (0.3357, -23.7196) (0.8395, -23.7154) (1.5617, -23.8775) (1.79, -23.9806) knots 0 0 0 1 2 2 2
  line L206 (1.79, -23.9806) -> (1.7977, -24.9184)
  line L207 (1.7977, -24.9184) -> (1.6927, -24.9192)
  spline S141 degree 2 poles (1.6927, -24.9192) (1.4535, -24.7707) (0.8114, -24.552) (0.5454, -24.5542) knots 0 0 0 1 2 2 2
  spline S142 degree 2 poles (0.5454, -24.5542) (0.388, -24.5555) (0.021, -24.6145) (-0.1042, -24.7065) knots 0 0 0 1 2 2 2
  spline S143 degree 2 poles (-0.1042, -24.7065) (-0.2016, -24.7808) (-0.3188, -24.9952) (-0.3172, -25.1876) knots 0 0 0 1 2 2 2
  spline S144 degree 2 poles (-0.3172, -25.1876) (-0.3156, -25.3801) (-0.146, -25.5851) (-0.0056, -25.633) knots 0 0 0 1 2 2 2
  spline S145 degree 2 poles (-0.0056, -25.633) (0.1347, -25.6808) (0.5232, -25.6881) (0.6737, -25.6869) knots 0 0 0 1 2 2 2
  line L208 (0.6737, -25.6869) -> (0.8591, -25.6854)
  line L209 (0.8591, -25.6854) -> (0.8653, -26.4447)
  line L210 (0.8653, -26.4447) -> (0.6939, -26.4461)
  spline S146 degree 2 poles (0.6939, -26.4461) (0.4979, -26.4477) (0.1658, -26.4854) (0.0508, -26.5388) knots 0 0 0 1 2 2 2
  spline S147 degree 2 poles (0.0508, -26.5388) (-0.0642, -26.5958) (-0.1921, -26.7928) (-0.1907, -26.9607) knots 0 0 0 1 2 2 2
  spline S148 degree 2 poles (-0.1907, -26.9607) (-0.1896, -27.0937) (-0.0658, -27.2572) (0.022, -27.3019) knots 0 0 0 1 2 2 2
  spline S149 degree 2 poles (0.022, -27.3019) (0.1274, -27.3536) (0.4076, -27.3863) (0.5056, -27.3855) knots 0 0 0 1 2 2 2
  spline S150 degree 2 poles (0.5056, -27.3855) (0.6631, -27.3842) (0.9949, -27.308) (1.1483, -27.2472) knots 0 0 0 1 2 2 2
  spline S151 degree 2 poles (1.1483, -27.2472) (1.2704, -27.2007) (1.5352, -27.0516) (1.5978, -27.0126) knots 0 0 0 1 2 2 2
  line L211 (1.5978, -27.0126) -> (1.6888, -27.0119)
  line L212 (1.6888, -27.0119) -> (1.6964, -27.9356)
  spline S152 degree 2 poles (1.6964, -27.9356) (1.4732, -28.0319) (0.7189, -28.2165) (0.3235, -28.2198) knots 0 0 0 1 2 2 2
  spline S153 degree 2 poles (0.3235, -28.2198) (-0.0614, -28.2229) (-0.6294, -28.0946) (-0.8299, -27.9668) knots 0 0 0 1 2 2 2
  spline S154 degree 2 poles (-0.8299, -27.9668) (-1.0514, -27.8321) (-1.2753, -27.414) (-1.2775, -27.1516) knots 0 0 0 1 2 2 2
  spline S155 degree 2 poles (-1.2775, -27.1516) (-1.2805, -26.7807) (-0.8581, -26.2243) (-0.5089, -26.141) knots 0 0 0 1 2 2 2
  line L213 (-0.5089, -26.141) -> (-0.5092, -26.099)
  spline S156 degree 2 poles (-0.5092, -26.099) (-0.6633, -26.0793) (-0.9582, -25.9697) (-1.0992, -25.8449) knots 0 0 0 1 2 2 2
  spline S157 degree 2 poles (-1.0992, -25.8449) (-1.2296, -25.734) (-1.4039, -25.3785) (-1.4059, -25.1335) knots 0 0 0 1 2 2 2
  line L214 (-3.122, -23.6125) -> (-2.1029, -23.725)
  line L215 (-2.1029, -23.725) -> (-2.2282, -24.8589)
  line L216 (-2.2282, -24.8589) -> (-3.2472, -24.7463)
  line L217 (-3.2472, -24.7463) -> (-3.122, -23.6125)
  spline S158 degree 2 poles (-7.4957, -24.9219) (-7.3691, -24.3765) (-7.0053, -23.5989) (-6.7469, -23.3679) knots 0 0 0 1 2 2 2
  spline S159 degree 2 poles (-6.7469, -23.3679) (-6.4927, -23.1396) (-5.8108, -23.0033) (-5.3677, -23.1062) knots 0 0 0 1 2 2 2
  spline S160 degree 2 poles (-5.3677, -23.1062) (-4.9212, -23.2099) (-4.3726, -23.6319) (-4.2432, -23.9565) knots 0 0 0 1 2 2 2
  spline S161 degree 2 poles (-4.2432, -23.9565) (-4.1131, -24.2777) (-4.1276, -25.1293) (-4.2543, -25.6747) knots 0 0 0 1 2 2 2
  spline S162 degree 2 poles (-4.2543, -25.6747) (-4.3841, -26.2337) (-4.7416, -26.9841) (-5.0057, -27.2245) knots 0 0 0 1 2 2 2
  spline S163 degree 2 poles (-5.0057, -27.2245) (-5.2683, -27.458) (-5.9554, -27.5859) (-6.3849, -27.4861) knots 0 0 0 1 2 2 2
  spline S164 degree 2 poles (-6.3849, -27.4861) (-6.8382, -27.3809) (-7.3784, -26.9537) (-7.507, -26.6256) knots 0 0 0 1 2 2 2
  spline S165 degree 2 poles (-7.507, -26.6256) (-7.6338, -26.3052) (-7.6184, -25.4502) (-7.4957, -24.9219) knots 0 0 0 1 2 2 2
  spline S166 degree 2 poles (-6.4357, -25.1681) (-6.617, -25.9486) (-6.5078, -26.6386) (-6.2044, -26.709) knots 0 0 0 1 2 2 2
  spline S167 degree 2 poles (-6.2044, -26.709) (-5.9011, -26.7794) (-5.4956, -26.209) (-5.3135, -25.4251) knots 0 0 0 1 2 2 2
  spline S168 degree 2 poles (-5.3135, -25.4251) (-5.1346, -24.6548) (-5.2449, -23.9538) (-5.5482, -23.8834) knots 0 0 0 1 2 2 2
  spline S169 degree 2 poles (-5.5482, -23.8834) (-5.8482, -23.8137) (-6.256, -24.3943) (-6.4357, -25.1681) knots 0 0 0 1 2 2 2
  line L218 (-10.0679, -26.4735) -> (-9.2898, -24.9435)
  line L219 (-9.2898, -24.9435) -> (-8.7348, -25.1576)
  line L220 (-8.7348, -25.1576) -> (-9.1865, -26.8137)
  line L221 (-9.1865, -26.8137) -> (-10.0679, -26.4735)
  line L222 (-11.2072, -26.0338) -> (-10.4291, -24.5037)
  line L223 (-10.4291, -24.5037) -> (-9.8741, -24.7179)
  line L224 (-9.8741, -24.7179) -> (-10.3258, -26.374)
  line L225 (-10.3258, -26.374) -> (-11.2072, -26.0338)
  line L226 (-17.2727, -22.2933) -> (-13.6428, -19.5238)
  line L227 (-13.6428, -19.5238) -> (-12.7024, -20.1508)
  line L228 (-12.7024, -20.1508) -> (-13.8635, -24.5665)
  line L229 (-13.8635, -24.5665) -> (-14.798, -23.9434)
  line L230 (-14.798, -23.9434) -> (-13.9564, -20.9844)
  line L231 (-13.9564, -20.9844) -> (-16.3614, -22.9009)
  line L232 (-16.3614, -22.9009) -> (-17.2727, -22.2933)
  spline S170 degree 2 poles (-20.2255, -16.3773) (-19.8138, -15.9978) (-19.0754, -15.5599) (-18.7318, -15.5145) knots 0 0 0 1 2 2 2
  spline S171 degree 2 poles (-18.7318, -15.5145) (-18.3931, -15.4689) (-17.7529, -15.7402) (-17.4446, -16.0747) knots 0 0 0 1 2 2 2
  spline S172 degree 2 poles (-17.4446, -16.0747) (-17.134, -16.4118) (-16.9181, -17.0694) (-16.9939, -17.4105) knots 0 0 0 1 2 2 2
  spline S173 degree 2 poles (-16.9939, -17.4105) (-17.0672, -17.7492) (-17.5587, -18.4449) (-17.9703, -18.8243) knots 0 0 0 1 2 2 2
  spline S174 degree 2 poles (-17.9703, -18.8243) (-18.3923, -19.2132) (-19.1102, -19.6321) (-19.4639, -19.6821) knots 0 0 0 1 2 2 2
  spline S175 degree 2 poles (-19.4639, -19.6821) (-19.8125, -19.7273) (-20.4523, -19.4461) (-20.7511, -19.1219) knots 0 0 0 1 2 2 2
  spline S176 degree 2 poles (-20.7511, -19.1219) (-21.0665, -18.7797) (-21.2724, -18.1225) (-21.194, -17.779) knots 0 0 0 1 2 2 2
  spline S177 degree 2 poles (-21.194, -17.779) (-21.1184, -17.4428) (-20.6244, -16.7448) (-20.2255, -16.3773) knots 0 0 0 1 2 2 2
  spline S178 degree 2 poles (-19.488, -17.1775) (-20.0773, -17.7205) (-20.3754, -18.3522) (-20.1644, -18.5812) knots 0 0 0 1 2 2 2
  spline S179 degree 2 poles (-20.1644, -18.5812) (-19.9533, -18.8103) (-19.2971, -18.5671) (-18.7053, -18.0217) knots 0 0 0 1 2 2 2
  spline S180 degree 2 poles (-18.7053, -18.0217) (-18.1238, -17.4857) (-17.8202, -16.8444) (-18.0313, -16.6154) knots 0 0 0 1 2 2 2
  spline S181 degree 2 poles (-18.0313, -16.6154) (-18.24, -16.3889) (-18.9039, -16.6392) (-19.488, -17.1775) knots 0 0 0 1 2 2 2
  spline S182 degree 2 poles (-21.7836, -12.411) (-21.5533, -12.2581) (-21.0262, -12.1854) (-20.7585, -12.2722) knots 0 0 0 1 2 2 2
  spline S183 degree 2 poles (-20.7585, -12.2722) (-20.4908, -12.3591) (-19.9772, -12.7784) (-19.7508, -13.1195) knots 0 0 0 1 2 2 2
  spline S184 degree 2 poles (-19.7508, -13.1195) (-19.5088, -13.4839) (-19.3131, -14.1393) (-19.3398, -14.4091) knots 0 0 0 1 2 2 2
  spline S185 degree 2 poles (-19.3398, -14.4091) (-19.3684, -14.6759) (-19.6477, -15.0966) (-19.8635, -15.2398) knots 0 0 0 1 2 2 2
  spline S186 degree 2 poles (-19.8635, -15.2398) (-20.1725, -15.445) (-20.81, -15.3768) (-21.1618, -15.1442) knots 0 0 0 1 2 2 2
  line L233 (-21.1618, -15.1442) -> (-21.1764, -15.1538)
  spline S187 degree 2 poles (-21.1764, -15.1538) (-21.1199, -15.5742) (-21.3937, -16.1171) (-21.6648, -16.2971) knots 0 0 0 1 2 2 2
  spline S188 degree 2 poles (-21.6648, -16.2971) (-21.863, -16.4288) (-22.3261, -16.4842) (-22.5773, -16.4031) knots 0 0 0 1 2 2 2
  spline S189 degree 2 poles (-22.5773, -16.4031) (-22.8188, -16.3241) (-23.311, -15.9243) (-23.5201, -15.6094) knots 0 0 0 1 2 2 2
  spline S190 degree 2 poles (-23.5201, -15.6094) (-23.7407, -15.2771) (-23.9269, -14.6867) (-23.9167, -14.4489) knots 0 0 0 1 2 2 2
  spline S191 degree 2 poles (-23.9167, -14.4489) (-23.9085, -14.2082) (-23.6865, -13.8088) (-23.4912, -13.6791) knots 0 0 0 1 2 2 2
  spline S192 degree 2 poles (-23.4912, -13.6791) (-23.2346, -13.5088) (-22.6262, -13.5333) (-22.2801, -13.7445) knots 0 0 0 1 2 2 2
  line L234 (-22.2801, -13.7445) -> (-22.2684, -13.7368)
  spline S193 degree 2 poles (-22.2684, -13.7368) (-22.3607, -13.2814) (-22.113, -12.6297) (-21.7836, -12.411) knots 0 0 0 1 2 2 2
  spline S194 degree 2 poles (-21.1534, -13.2779) (-21.3313, -13.396) (-21.4172, -13.6714) (-21.3741, -13.9957) knots 0 0 0 1 2 2 2
  spline S195 degree 2 poles (-21.3741, -13.9957) (-21.3597, -14.0869) (-21.2856, -14.4199) (-21.2616, -14.551) knots 0 0 0 1 2 2 2
  spline S196 degree 2 poles (-21.2616, -14.551) (-21.1064, -14.5823) (-20.7278, -14.5452) (-20.5617, -14.4349) knots 0 0 0 1 2 2 2
  spline S197 degree 2 poles (-20.5617, -14.4349) (-20.311, -14.2684) (-20.2236, -13.7484) (-20.3959, -13.489) knots 0 0 0 1 2 2 2
  spline S198 degree 2 poles (-20.3959, -13.489) (-20.4443, -13.4161) (-20.6109, -13.2663) (-20.704, -13.2273) knots 0 0 0 1 2 2 2
  spline S199 degree 2 poles (-20.704, -13.2273) (-20.8116, -13.1854) (-21.0252, -13.1927) (-21.1534, -13.2779) knots 0 0 0 1 2 2 2
  spline S200 degree 2 poles (-22.8036, -14.4869) (-22.9873, -14.6089) (-23.0453, -14.996) (-22.9079, -15.203) knots 0 0 0 1 2 2 2
  spline S201 degree 2 poles (-22.9079, -15.203) (-22.7763, -15.4012) (-22.4174, -15.5115) (-22.2716, -15.4148) knots 0 0 0 1 2 2 2
  spline S202 degree 2 poles (-22.2716, -15.4148) (-22.1288, -15.3199) (-22.0477, -15.0561) (-22.0774, -14.8532) knots 0 0 0 1 2 2 2
  spline S203 degree 2 poles (-22.0774, -14.8532) (-22.087, -14.7629) (-22.138, -14.528) (-22.1822, -14.3348) knots 0 0 0 1 2 2 2
  spline S204 degree 2 poles (-22.1822, -14.3348) (-22.3666, -14.3228) (-22.655, -14.3882) (-22.8036, -14.4869) knots 0 0 0 1 2 2 2
  dimension "d142" = 47.625
  constraints: 1 centre point, 1 coincident, 1 other
  measures "d142" diameter of A0
extrude "Extrusion18" cut sketch "Sketch24" against normal blind 1.905